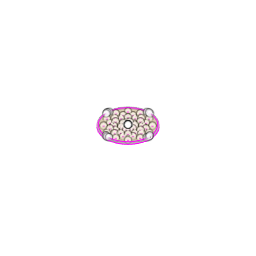
Gyro Shell Top Print rev 0.1 (Autodesk Fusion 360 design; units mm, degrees)
Autodesk Fusion 360 part; units mm, degrees
sketch "sketch 676" plane through (0, 0, 5.4839) normal (0, 0, 1) x (1, 0, 0)
  circle A0 centre (0, 0) radius 57.0059
extrude "Extrude1" add sketch "sketch 676" along normal blind 3.81
hole "Hole1" at (0.3032, 54.1442, 9.2939) direction (0, 0, -1) diameter 2.032 depth 10.16 tip angle 118 counterbore diameter 4.064 counterbore depth 2.032
pattern_circular "C-Pattern1" count 4 over 360 about axis through (0, 0, -205.75) along (0, 0, 1) of "Hole1"
sketch "sketch 690" plane through (0, 0, 9.2939) normal (0, 0, 1) x (-1, 0, 0)
  arc A0 (2.3233, -53.1911) -> (3.6016, -54.0251) centre (3.5171, -52.7579) ccw
  arc A1 (3.6016, -54.0251) -> (53.9814, -4.2063) centre (0, 0) ccw
  arc A2 (3.6016, -54.0251) -> (53.9814, -4.2063) centre (0, 0) ccw
  arc A3 (53.9814, -4.2063) -> (53.1618, -2.9188) centre (52.7152, -4.1077) ccw
  arc A4 (53.1911, 2.3233) -> (53.1618, -2.9188) centre (54.1442, -0.3032) ccw
  arc A5 (53.1911, 2.3233) -> (54.0251, 3.6016) centre (52.7579, 3.5171) ccw
  arc A6 (54.0251, 3.6016) -> (4.2063, 53.9814) centre (0, 0) ccw
  arc A7 (54.0251, 3.6016) -> (4.2063, 53.9814) centre (0, 0) ccw
  arc A8 (4.2063, 53.9814) -> (2.9188, 53.1618) centre (4.1077, 52.7152) ccw
  arc A9 (-2.3233, 53.1911) -> (2.9188, 53.1618) centre (0.3032, 54.1442) ccw
  arc A10 (-2.3233, 53.1911) -> (-3.6016, 54.0251) centre (-3.5171, 52.7579) ccw
  arc A11 (-3.6016, 54.0251) -> (-53.9814, 4.2063) centre (0, 0) ccw
  arc A12 (-3.6016, 54.0251) -> (-53.9814, 4.2063) centre (0, 0) ccw
  arc A13 (-53.9814, 4.2063) -> (-53.1618, 2.9188) centre (-52.7152, 4.1077) ccw
  arc A14 (-53.1911, -2.3233) -> (-53.1618, 2.9188) centre (-54.1442, 0.3032) ccw
  arc A15 (-53.1911, -2.3233) -> (-54.0251, -3.6016) centre (-52.7579, -3.5171) ccw
  arc A16 (-54.0251, -3.6016) -> (-4.2063, -53.9814) centre (0, 0) ccw
  arc A17 (-54.0251, -3.6016) -> (-4.2063, -53.9814) centre (0, 0) ccw
  arc A18 (-4.2063, -53.9814) -> (-2.9188, -53.1618) centre (-4.1077, -52.7152) ccw
  arc A19 (2.3233, -53.1911) -> (-2.9188, -53.1618) centre (-0.3032, -54.1442) ccw
extrude "Extrude2" cut sketch "sketch 690" against normal blind 2.54
sketch "sketch 791" plane through (0, 0, 6.7539) normal (0, 0, 1) x (-1, 0, 0)
  circle A0 centre (10.9985, -6.35) radius 1.905
  circle A1 centre (10.9985, 6.35) radius 1.905
  circle A2 centre (0, 12.7) radius 1.905
  circle A3 centre (-10.9985, 6.35) radius 1.905
  circle A4 centre (-10.9985, -6.35) radius 1.905
  circle A5 centre (0, -12.7) radius 1.905
  circle A6 centre (-18.5941, -18.5941) radius 1.905
  circle A7 centre (6.8059, -25.4) radius 1.905
  circle A8 centre (25.4, -6.8059) radius 1.905
  circle A9 centre (-25.4, 6.8059) radius 1.905
  circle A10 centre (18.5941, 18.5941) radius 1.905
  circle A11 centre (6.8059, 25.4) radius 1.905
  circle A12 centre (-17.145, 29.696) radius 1.905
  circle A13 centre (-34.29, 0) radius 1.905
  circle A14 centre (-17.145, -29.696) radius 1.905
  circle A15 centre (17.145, -29.696) radius 1.905
  circle A16 centre (34.29, 0) radius 1.905
  circle A17 centre (29.696, 17.145) radius 1.905
  circle A18 centre (11.57, 43.18) radius 1.905
  circle A19 centre (-31.61, 31.61) radius 1.905
  circle A20 centre (-43.18, -11.57) radius 1.905
  circle A21 centre (-11.57, -43.18) radius 1.905
  circle A22 centre (31.61, -31.61) radius 1.905
  circle A23 centre (43.18, 11.57) radius 1.905
  circle A24 centre (43.18, -11.57) radius 1.905
  circle A25 centre (11.57, -43.18) radius 1.905
  circle A26 centre (-31.61, -31.61) radius 1.905
  circle A27 centre (-43.18, 11.57) radius 1.905
  circle A28 centre (-11.57, 43.18) radius 1.905
  circle A29 centre (31.61, 31.61) radius 1.905
  circle A30 centre (17.145, 29.696) radius 1.905
  circle A31 centre (29.696, -17.145) radius 1.905
  circle A32 centre (0, -34.29) radius 1.905
  circle A33 centre (-29.696, -17.145) radius 1.905
  circle A34 centre (-29.696, 17.145) radius 1.905
  circle A35 centre (0, 34.29) radius 1.905
  circle A36 centre (-6.8059, 25.4) radius 1.905
  circle A37 centre (-18.5941, 18.5941) radius 1.905
  circle A38 centre (25.4, 6.8059) radius 1.905
  circle A39 centre (18.5941, -18.5941) radius 1.905
  circle A40 centre (-6.8059, -25.4) radius 1.905
  circle A41 centre (-25.4, -6.8059) radius 1.905
  circle A42 centre (-6.35, -10.9985) radius 1.905
  circle A43 centre (-12.7, 0) radius 1.905
  circle A44 centre (-6.35, 10.9985) radius 1.905
  circle A45 centre (6.35, 10.9985) radius 1.905
  circle A46 centre (12.7, 0) radius 1.905
  circle A47 centre (6.35, -10.9985) radius 1.905
extrude "Extrude3" cut sketch "sketch 791" against normal blind 5.08
